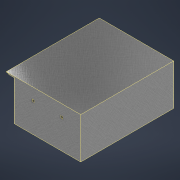
# Autodesk Inventor part: McCrea_zadne_oko_walle
Saved by Autodesk Inventor 2022 (Build 260153000, 153)
## iProperties
Created: 2022-01-17
Part Number: McCrea_zadne_oko_walle
Material: Silver
Document SubType Name: Modeling
Designer: student
Density: 10.49 g/cm^3
Appearance: Silver
Author: student
Autodesk Inventor part; units mm, degrees
ref_plane "YZ Plane" through (0, 0, 0) normal (1, 0, 0) x (0, 1, 0)
ref_plane "XZ Plane" through (0, 0, 0) normal (0, 1, 0) x (-1, 0, 0)
ref_plane "XY Plane" through (0, 0, 0) normal (0, 0, 1) x (1, 0, 0)
sketch "Sketch1" plane through (0, 0, 0) normal (0, 0, 1) x (1, 0, 0)
  line L0 (-23.6052, 15.8968) -> (1.3948, 15.8968)
  line L1 (1.3948, 15.8968) -> (1.3948, 0.4466)
  line L2 (1.3948, 0.4466) -> (-23.6052, 0.4466)
  line L3 (-23.6052, 0.4466) -> (-23.6052, 15.4466)
  line L4 (-23.6052, 15.8968) -> (-26.1052, 15.8968)
  line L5 (-25.6052, 15.7466) -> (-25.6052, 15.4466)
  line L6 (-25.6052, 15.4466) -> (-23.6052, 15.4466)
  line L7 (-26.1052, 15.8968) -> (-26.6052, 15.8968)
  line L8 (-26.6052, 15.8968) -> (-26.6052, 15.7466)
  line L9 (-26.6052, 15.7466) -> (-25.6052, 15.7466)
  point P0 (0, 0)
  dimension "d0" = 15
  dimension "d1" = 25
  dimension "d2" = 2
  dimension "d3" = 1
  dimension "d4" = 2.5
  dimension "d5" = 0.5
  dimension "d6" = 0.1502
  dimension "d7" = 0.3
  constraints: 20 end point, 5 perpendicular, 3 horizontal, 2 parallel
  measures "d0" distance of L2.end L3.end
  measures "d1" distance of L1.end L2.end
  measures "d2" distance of L5.end L3.end
  measures "d3" distance of L8.end L5.start
  measures "d4" distance of L0.start L4.end
  measures "d5" distance of L4.end L7.end
  measures "d6" distance of L7.end L8.end
  measures "d7" distance of L5.start L5.end
extrude "Extrusion1" add sketch "Sketch1" along normal blind 35
sketch "Sketch4" plane through (0, 0, 35) normal (0, 0, 1) x (1, 0, 0)
  line L0 (-26.6052, 15.8968) -> (-26.6052, 15.7466) projected
  line L1 (-26.6052, 15.7466) -> (-25.6052, 15.7466) projected
  line L2 (-25.6052, 15.7466) -> (-25.6052, 15.4466) projected
  line L3 (-25.6052, 15.4466) -> (-23.6052, 15.4466) projected
  line L4 (-23.6052, 15.4466) -> (-23.6052, 0.4466) projected
  line L5 (-23.6052, 0.4466) -> (1.3948, 0.4466) projected
  line L6 (1.3948, 0.4466) -> (1.3948, 15.8968) projected
  line L7 (1.3948, 15.8968) -> (-26.6052, 15.8968) projected
  line L8 (-16.9052, 11.8968) -> (-16.1052, 11.8968)
  line L9 (-16.1052, 11.8968) -> (-16.1052, 11.0968)
  line L10 (-16.1052, 11.0968) -> (-16.9052, 11.0968)
  line L11 (-16.9052, 11.0968) -> (-16.9052, 11.8968)
  line L12 (-23.6052, 0.4466) -> (1.3948, 0.4466) projected
  line L13 (-11.1052, 0.4466) -> (-11.1052, 15.8968)
  line L14 (1.3948, 15.8968) -> (-26.6052, 15.8968) projected
  line L15 (-5.3052, 11.8968) -> (-6.1052, 11.8968)
  line L16 (-6.1052, 11.8968) -> (-6.1052, 11.0968)
  line L17 (-6.1052, 11.0968) -> (-5.3052, 11.0968)
  line L18 (-5.3052, 11.0968) -> (-5.3052, 11.8968)
  point P0 (0, 0)
  dimension "d26" = 10
  dimension "d27" = 0.8
  dimension "d28" = 0.8
  dimension "d29" = 4
  constraints: 18 end point, 4 symmetric about line, 2 parallel, 2 perpendicular, 1 horizontal, 1 midpoint, 1 point on line
  measures "d26" diameter of L9 L13
  measures "d27" distance of L9.end L10.end
  measures "d28" distance of L8.end L9.end
  measures "d29" distance between parallel lines of L7 L8
extrude "Extrusion2" cut sketch "Sketch4" against normal blind 1 contours L8 L9 L10 L11 | L18 L17 L16 L15
sketch "Sketch5" plane through (-23.6052, 0.4466, 0) normal (-1, 0, 0) x (0, 0, 1)
  line L0 (0, 15) -> (0, 0) projected
  line L1 (0, 0) -> (35, 0) projected
  line L2 (35, 15) -> (35, 0) projected
  line L3 (0, 15) -> (35, 15) projected
  line L4 (12, 5) -> (15, 5)
  line L5 (15, 5) -> (15, 4)
  line L6 (15, 4) -> (12, 4)
  line L7 (12, 4) -> (12, 5)
  point P0 (0, -0.4466)
  dimension "d32" = 1
  dimension "d33" = 3
  dimension "d34" = 10
  dimension "d35" = 20
  constraints: 8 end point, 2 parallel, 1 horizontal, 1 perpendicular
  measures "d32" distance between parallel lines of L4 L6
  measures "d33" distance of L4.start L4.end
  measures "d34" distance between parallel lines of L3 L4
  measures "d35" distance between parallel lines of L2 L5
extrude "Extrusion3" cut sketch "Sketch5" against normal blind 1 contours L4 L5 L6 L7
equation "\"d28\" = d27"
body "Solid1"
